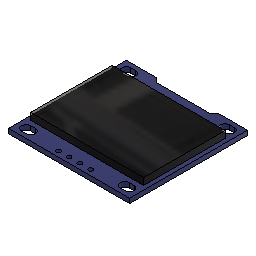
key_emulator (Autodesk Fusion 360 archive; units mm, degrees)
design "OLED Display"
Autodesk Fusion 360 part; units mm, degrees
sketch "Sketch1" plane through (0, 0, 0) normal (0, 1, 0) x (1, 0, 0)
  line L0 (14.25, -13.875) -> (-14.25, -13.875)
  line L1 (-14.25, -13.875) -> (-14.25, 13.875)
  line L2 (14.25, 13.875) -> (14.25, -13.875)
  line L3 (14.25, -13.875) -> (-14.25, 13.875) construction
  line L4 (-14.25, -13.875) -> (14.25, 13.875) construction
  line L5 (-7.25, 13.875) -> (-6.25, 12.875)
  line L6 (-6.25, 12.875) -> (6.25, 12.875)
  line L7 (6.25, 12.875) -> (7.25, 13.875)
  line L8 (-14.25, 13.875) -> (-7.25, 13.875)
  line L9 (7.25, 13.875) -> (14.25, 13.875)
  line L10 (-13.25, -10.725) -> (-10, -10.725)
  line L11 (-10, -10.725) -> (-10, -12.875)
  line L12 (-10, -12.875) -> (-13.25, -12.875)
  line L13 (-13.25, -12.875) -> (-13.25, -10.725)
  line L14 (0, 0) -> (0, -13.875) construction
  line L15 (0, 0) -> (14.25, 0) construction
  line L16 (13.25, -10.725) -> (10, -10.725)
  line L17 (10, -10.725) -> (10, -12.875)
  line L18 (10, -12.875) -> (13.25, -12.875)
  line L19 (13.25, -12.875) -> (13.25, -10.725)
  line L20 (-13.25, 10.725) -> (-10, 10.725)
  line L21 (-10, 12.875) -> (-13.25, 12.875)
  line L22 (10, 12.875) -> (13.25, 12.875)
  line L23 (-13.25, 12.875) -> (-13.25, 10.725)
  line L24 (10, 10.725) -> (10, 12.875)
  line L25 (13.25, 10.725) -> (10, 10.725)
  line L26 (-10, 10.725) -> (-10, 12.875)
  line L27 (13.25, 12.875) -> (13.25, 10.725)
  dimension "d1" = 28.5
  dimension "d2" = 27.75
  dimension "d3" = 135
  dimension "d4" = 7
  dimension "d5" = 7
  dimension "d6" = 1
  dimension "d7" = 3.25
  dimension "d8" = 2.15
  dimension "d9" = 1
  dimension "d10" = 1
  constraint horizontal L0
  constraint perpendicular L0 L1
  constraint parallel L0 L8
  constraint parallel L1 L2
  constraint coincident L3 L14.start
  constraint coincident L4 L14.start
  constraint coincident L14.start L15.start
  constraint parallel L6 L8
  constraint coincident L7.end L8
  constraint perpendicular L5 L7
  constraint collinear L8 L9
  constraint horizontal L10
  constraint vertical L11
  constraint horizontal L12
  constraint vertical L13
  constraint midpoint L0 L14.end
  constraint midpoint L2 L15.end
  constraint symmetric L10.start L14 L16.start
  constraint symmetric L10.end L14 L16.end
  constraint symmetric L11.end L14 L17.end
  constraint symmetric L12.end L14 L18.end
  constraint symmetric L10.start L15 L20.start
  constraint symmetric L10.end L15 L20.end
  constraint symmetric L11.end L15 L21.start
  constraint symmetric L12.end L15 L21.end
  constraint symmetric L15 L17.end L22.start
  constraint symmetric L15 L16.start L25.start
  constraint symmetric L15 L16.end L24.start
  constraint symmetric L15 L18.end L22.end
  measures "d1" distance of L1.end L2.start
  measures "d2" distance of L0.end L1.end
  measures "d3" angle of L5 L6
  measures "d4" distance of L1.end L5.start
  measures "d5" distance of L2.start L7.end
  measures "d6" horizontal distance of L6.end L7.end
  measures "d7" distance of L10.start L10.end
  measures "d8" distance of L10.start L12.end
  measures "d9" distance of L0 L12
  measures "d10" distance of L1 L13
extrude "Extrude1" add sketch "Sketch1" along normal blind 1.1 makes body 1
fillet "Fillet1" radius 1.075 16 edges at (13.25, 0.55, -12.875) (13.25, 0.55, -10.725) (10, 0.55, -10.725) (10, 0.55, -12.875) (-13.25, 0.55, -12.875) (-13.25, 0.55, -10.725) (-10, 0.55, -10.725) (-10, 0.55, -12.875) (-10, 0.55, 10.725) (-13.25, 0.55, 10.725) (-13.25, 0.55, 12.875) (-10, 0.55, 12.875) (13.25, 0.55, 12.875) (10, 0.55, 12.875) (10, 0.55, 10.725) (13.25, 0.55, 10.725) on bodies 1
sketch "Sketch2" plane through (0, 1.1, 0) normal (0, 1, 0) x (-1, 0, 0)
  arc A0 (-12.175, 12.875) -> (-12.175, 10.725) centre (-12.175, 11.8) ccw
  line L0 (-12.175, 12.875) -> (-11.075, 12.875)
  arc A1 (-11.075, 10.725) -> (-11.075, 12.875) centre (-11.075, 11.8) ccw
  line L1 (-11.075, 10.725) -> (-12.175, 10.725)
  line L2 (-11.075, -12.875) -> (-12.175, -12.875)
  arc A2 (-12.175, -10.725) -> (-12.175, -12.875) centre (-12.175, -11.8) ccw
  line L3 (-12.175, -10.725) -> (-11.075, -10.725)
  arc A3 (-11.075, -12.875) -> (-11.075, -10.725) centre (-11.075, -11.8) ccw
  line L4 (11.075, 12.875) -> (12.175, 12.875)
  arc A4 (12.175, 10.725) -> (12.175, 12.875) centre (12.175, 11.8) ccw
  line L5 (12.175, 10.725) -> (11.075, 10.725)
  arc A5 (11.075, 12.875) -> (11.075, 10.725) centre (11.075, 11.8) ccw
  arc A6 (11.075, -10.725) -> (11.075, -12.875) centre (11.075, -11.8) ccw
  line L6 (11.075, -10.725) -> (12.175, -10.725)
  arc A7 (12.175, -12.875) -> (12.175, -10.725) centre (12.175, -11.8) ccw
  line L7 (12.175, -12.875) -> (11.075, -12.875)
  line L8 (-7.25, -13.875) -> (-6.25, -12.875)
  line L9 (-6.25, -12.875) -> (6.25, -12.875)
  line L10 (6.25, -12.875) -> (7.25, -13.875)
  line L11 (7.25, -13.875) -> (14.25, -13.875)
  line L12 (14.25, -13.875) -> (14.25, 13.875)
  line L13 (14.25, 13.875) -> (-14.25, 13.875)
  line L14 (-14.25, 13.875) -> (-14.25, -13.875)
  line L15 (-14.25, -13.875) -> (-7.25, -13.875)
  line L16 (-13.3, 9.625) -> (13.3, 9.625)
  line L17 (13.3, 9.625) -> (13.3, -9.575)
  line L18 (13.3, -9.575) -> (-13.3, -9.575)
  line L19 (-13.3, -9.575) -> (-13.3, 9.625)
  line L20 (-13.3, 9.625) -> (13.3, -9.575) construction
  line L21 (13.3, 9.625) -> (-13.3, -9.575) construction
  point P0 (0, 0.025)
  dimension "d14" = 26.6
  dimension "d15" = 19.2
  dimension "d16" = 4.25
  constraint horizontal L16
  constraint perpendicular L16 L17
  constraint parallel L16 L18
  constraint parallel L17 L19
  constraint coincident L20 P0
  constraint coincident L21 P0
  constraint vertical origin P0
  measures "d14" distance of L17.end L18.end
  measures "d15" distance of L16.end L17.end
  measures "d16" distance of L13 L16
extrude "Extrude2" add sketch "Sketch2" along normal blind 1.6 separate body contours L16 L17 L18 L19 makes body 2
sketch "Sketch3" plane through (0, 1.1, 0) normal (0, 1, 0) x (-1, 0, 0)
  arc A0 (-12.175, 12.875) -> (-12.175, 10.725) centre (-12.175, 11.8) ccw
  line L0 (-12.175, 12.875) -> (-11.075, 12.875)
  arc A1 (-11.075, 10.725) -> (-11.075, 12.875) centre (-11.075, 11.8) ccw
  line L1 (-11.075, 10.725) -> (-12.175, 10.725)
  line L2 (-11.075, -12.875) -> (-12.175, -12.875)
  arc A2 (-12.175, -10.725) -> (-12.175, -12.875) centre (-12.175, -11.8) ccw
  line L3 (-12.175, -10.725) -> (-11.075, -10.725)
  arc A3 (-11.075, -12.875) -> (-11.075, -10.725) centre (-11.075, -11.8) ccw
  line L4 (11.075, 12.875) -> (12.175, 12.875)
  arc A4 (12.175, 10.725) -> (12.175, 12.875) centre (12.175, 11.8) ccw
  line L5 (12.175, 10.725) -> (11.075, 10.725)
  arc A5 (11.075, 12.875) -> (11.075, 10.725) centre (11.075, 11.8) ccw
  arc A6 (11.075, -10.725) -> (11.075, -12.875) centre (11.075, -11.8) ccw
  line L6 (11.075, -10.725) -> (12.175, -10.725)
  arc A7 (12.175, -12.875) -> (12.175, -10.725) centre (12.175, -11.8) ccw
  line L7 (12.175, -12.875) -> (11.075, -12.875)
  line L8 (-7.25, -13.875) -> (-6.25, -12.875)
  line L9 (-6.25, -12.875) -> (6.25, -12.875)
  line L10 (6.25, -12.875) -> (7.25, -13.875)
  line L11 (7.25, -13.875) -> (14.25, -13.875)
  line L12 (14.25, -13.875) -> (14.25, 13.875)
  line L13 (14.25, 13.875) -> (-14.25, 13.875)
  line L14 (-14.25, 13.875) -> (-14.25, -13.875)
  line L15 (-14.25, -13.875) -> (-7.25, -13.875)
  line L16 (5.08, 13.875) -> (2.54, 13.875) construction
  line L17 (2.54, 13.875) -> (2.54, 11.335) construction
  line L18 (2.54, 11.335) -> (5.08, 11.335) construction
  line L19 (5.08, 11.335) -> (5.08, 13.875) construction
  line L20 (5.08, 13.875) -> (2.54, 11.335) construction
  circle A8 centre (3.81, 12.605) radius 0.508
  circle A9 centre (1.27, 12.605) radius 0.508
  circle A10 centre (-1.27, 12.605) radius 0.508
  circle A11 centre (-3.81, 12.605) radius 0.508
  point P0 (0, 13.875)
  point P1 (5.08, 13.875)
  dimension "d28" = 2.54
  dimension "d29" = 2.54
  dimension "d30" = 2.54
  dimension "d31" = 1.016
  dimension "d34" = -7.62
  dimension "d35" = 0
  constraint midpoint L13 P0
  constraint coincident L13 P1
  constraint horizontal L16
  constraint vertical L17
  constraint horizontal L18
  constraint vertical L19
  constraint coincident P1 L16.start
  constraint midpoint L20 A8.centre
  measures "d28" distance of P1 L16.end
  measures "d29" distance of P1 L18.end
  measures "d30" distance of P0 L16.end
  measures "d31" diameter of A8
extrude "Extrude3" cut sketch "Sketch3" against normal through all contours A8 | A9 | A10 | A11 bodies 1
equation "d13 = ( 2.15 / 2 ) * 1 mm"
equation "d34 = ( -2.54 * 3 ) * 1 mm"

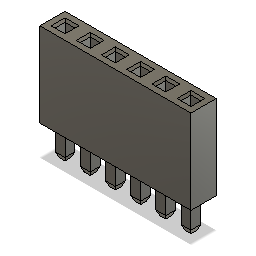
design "Pins"
Autodesk Fusion 360 part; units mm, degrees
sketch "Sketch1" plane through (0, 0, 0) normal (0, 1, 0) x (1, 0, 0)
  line L0 (0, 0) -> (15.24, 0)
  line L1 (15.24, 0) -> (15.24, -2.54)
  line L2 (15.24, -2.54) -> (0, -2.54)
  line L3 (0, -2.54) -> (0, 0)
  line L4 (0, 0) -> (2.54, -2.54) construction
  line L5 (0, 0) -> (3.5921, 0) construction
  line L6 (1.77, -0.77) -> (0.77, -0.77)
  line L7 (0.77, -0.77) -> (0.77, -1.77)
  line L8 (0.77, -1.77) -> (1.77, -1.77)
  line L9 (1.77, -1.77) -> (1.77, -0.77)
  line L10 (1.77, -0.77) -> (0.77, -1.77) construction
  line L11 (0.77, -0.77) -> (1.77, -1.77) construction
  line L12 (4.31, -0.77) -> (3.31, -0.77)
  line L13 (4.31, -0.77) -> (3.31, -1.77) construction
  line L14 (3.31, -1.77) -> (4.31, -1.77)
  line L15 (3.31, -0.77) -> (4.31, -1.77) construction
  line L16 (3.31, -0.77) -> (3.31, -1.77)
  line L17 (4.31, -1.77) -> (4.31, -0.77)
  line L18 (6.85, -0.77) -> (5.85, -0.77)
  line L19 (6.85, -0.77) -> (5.85, -1.77) construction
  line L20 (5.85, -1.77) -> (6.85, -1.77)
  line L21 (5.85, -0.77) -> (6.85, -1.77) construction
  line L22 (5.85, -0.77) -> (5.85, -1.77)
  line L23 (6.85, -1.77) -> (6.85, -0.77)
  line L24 (9.39, -0.77) -> (8.39, -0.77)
  line L25 (9.39, -0.77) -> (8.39, -1.77) construction
  line L26 (8.39, -1.77) -> (9.39, -1.77)
  line L27 (8.39, -0.77) -> (9.39, -1.77) construction
  line L28 (8.39, -0.77) -> (8.39, -1.77)
  line L29 (9.39, -1.77) -> (9.39, -0.77)
  line L30 (11.93, -0.77) -> (10.93, -0.77)
  line L31 (11.93, -0.77) -> (10.93, -1.77) construction
  line L32 (10.93, -1.77) -> (11.93, -1.77)
  line L33 (10.93, -0.77) -> (11.93, -1.77) construction
  line L34 (10.93, -0.77) -> (10.93, -1.77)
  line L35 (11.93, -1.77) -> (11.93, -0.77)
  line L36 (14.47, -0.77) -> (13.47, -0.77)
  line L37 (14.47, -0.77) -> (13.47, -1.77) construction
  line L38 (13.47, -1.77) -> (14.47, -1.77)
  line L39 (13.47, -0.77) -> (14.47, -1.77) construction
  line L40 (13.47, -0.77) -> (13.47, -1.77)
  line L41 (14.47, -1.77) -> (14.47, -0.77)
  point P0 (1.27, -1.27)
  point P1 (3.81, -1.27)
  point P2 (6.35, -1.27)
  point P3 (8.89, -1.27)
  point P4 (11.43, -1.27)
  point P5 (13.97, -1.27)
  dimension "d1" = 15.24
  dimension "d2" = 2.54
  dimension "d3" = 45
  dimension "d4" = 1
  dimension "d5" = 1
  dimension "d8" = 12.7
  dimension "d9" = 0
  constraint horizontal L0
  constraint vertical L1
  constraint horizontal L2
  constraint vertical L3
  constraint coincident L0.start L3.end
  constraint horizontal L5
  constraint coincident L2 L4.end
  constraint horizontal L6
  constraint perpendicular L6 L7
  constraint parallel L6 L8
  constraint parallel L7 L9
  constraint coincident L10 P0
  constraint coincident L11 P0
  constraint midpoint L4 P0
  measures "d1" distance of L1.end L2.end
  measures "d2" distance of L0.end L1.end
  measures "d3" angle of L4 L5
  measures "d4" distance of L7.end L8.end
  measures "d5" distance of L6.end L7.end
extrude "Extrude1" add sketch "Sketch1" along normal blind 8.5 makes body 1
chamfer "Chamfer1" distance 0.2 angle 45 4 edges at (1.77, 8.5, 1.27) (1.27, 8.5, 1.77) (0.77, 8.5, 1.27) (1.27, 8.5, 0.77) on bodies 1
pattern_linear "R-Pattern1" count 6 spacing 2.54 along (1, 0, 0) of "Chamfer1"
ref_plane "WorkPlane1" through (7.62, 4.25, 1.27) normal (0, 0, 1) x (1, 0, 0)
sketch "Sketch2" plane through (7.62, 4.25, 1.27) normal (0, 0, 1) x (1, 0, 0)
  line L0 (-5.85, 4.05) -> (-6.85, 4.05)
  line L1 (-6.85, 4.05) -> (-6.85, -4.25)
  line L2 (-6.85, -4.25) -> (-5.85, -4.25)
  line L3 (-5.85, -4.25) -> (-5.85, 4.05)
  line L4 (-6.85, -4.25) -> (-5.85, -4.25)
  line L5 (-5.85, -4.25) -> (-5.85, -7.25)
  line L6 (-5.85, -7.25) -> (-6.85, -7.25)
  line L7 (-6.85, -7.25) -> (-6.85, -4.25)
  line L8 (-6.85, -4.25) -> (-5.85, -4.25)
  line L9 (-5.85, -4.25) -> (-5.85, -2.75)
  line L10 (-5.85, -2.75) -> (-6.85, -2.75)
  line L11 (-6.85, -2.75) -> (-6.85, -4.25)
  dimension "d18" = 1
  dimension "d19" = 3
  dimension "d20" = 1.5
  constraint horizontal L4
  constraint vertical L5
  constraint horizontal L6
  constraint vertical L7
  constraint coincident L1.end L2.start
  constraint horizontal L8
  constraint vertical L9
  constraint horizontal L10
  constraint vertical L11
  constraint coincident L3 L9.end
  measures "d18" distance of L1.end L2.end
  measures "d19" distance of L1.end L6.end
  measures "d20" distance of L8 L10
extrude "Extrude2" add sketch "Sketch2" along normal mid plane 1 separate body contours L1 L2 L3 L4 L8 L9 L10 L11 | L2 L4 L5 L6 L7 L8 makes body 2
chamfer "Chamfer2" distance 0.5 distance2 0.2 3 edges at (1.27, -3, 1.77) (0.77, -3, 1.27) (1.27, -3, 0.77) measured on face at (1.4367, 0, 1.77) measured on face at (0.77, -1.5, 1.4367) measured on face at (1.4367, 0, 0.77) on bodies 2
chamfer "Chamfer3" distance 0.2 distance2 0.5 1 edges at (1.77, -3, 1.27) measured on face at (1.5033, -3, 1.17) on bodies 2
pattern_linear "R-Pattern2" count 6 spacing 2.54 along (1, 0, 0) of "Extrude2", "Chamfer2", "Chamfer3" makes body 3 at (3.9767, 0.1667, 1.77) makes body 4 at (6.5167, 0.1667, 1.77) makes body 5 at (8.7233, -1.1667, 0.77) makes body 6 at (11.5967, 0.1667, 1.77) makes body 7 at (14.1367, 0.1667, 1.77)
combine "Combine1" operation add target body 1 tool bodies 6 5 3 7 4 2
equation "d1 = ( 2.54 * 6 ) * 1 mm"
equation "d8 = ( 2.54 * 5 ) * 1 mm"
equation "d15 = ( 2.54 * 5 ) * 1 mm"
equation "d17 = ( -2.54 / 2 ) * 1 mm"
equation "d29 = ( 2.54 * 5 ) * 1 mm"

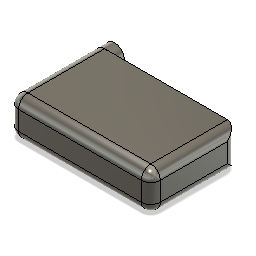
design "JJR 150mah battery"
Autodesk Fusion 360 part; units mm, degrees
sketch "Sketch1" plane through (0, 0, 0) normal (0, 1, 0) x (1, 0, 0)
  line L0 (14, -8.5) -> (-14, -8.5)
  line L1 (-14, -8.5) -> (-14, 8.5)
  line L2 (-14, 8.5) -> (14, 8.5)
  line L3 (14, 8.5) -> (14, -8.5)
  line L4 (14, -8.5) -> (-14, 8.5) construction
  line L5 (-14, -8.5) -> (14, 8.5) construction
  dimension "d1" = 28
  dimension "d2" = 17
  constraint horizontal L0
  constraint perpendicular L0 L1
  constraint parallel L0 L2
  constraint parallel L1 L3
  constraint coincident L4 origin
  constraint coincident L5 origin
  measures "d1" distance of L1.end L2.end
  measures "d2" distance of L0.end L1.end
extrude "Extrude1" add sketch "Sketch1" along normal blind 7.5 makes body 1
sketch "Sketch2" plane through (0, 0, -8.5) normal (0, 0, -1) x (-1, 0, 0)
  line L0 (-14, 0) -> (14, 0)
  line L1 (14, 0) -> (14, 7.5)
  line L2 (14, 7.5) -> (-14, 7.5)
  line L3 (-14, 7.5) -> (-14, 0)
  line L4 (14, 0) -> (6.5, 7.5) construction
  line L5 (14, 7.5) -> (6.5, 0) construction
  line L6 (14, 0) -> (10.25, 3.75) construction
  line L7 (10.25, 3.75) -> (14, 7.5) construction
  circle A0 centre (12.125, 5.625) radius 1.875
  circle A1 centre (12.125, 1.875) radius 1.875
  constraint coincident L0.end L1.start
  constraint coincident L2 L4.end
  constraint coincident L1.end L2.start
  constraint coincident L0 L5.end
  constraint vertical L4.end L5.end
  constraint perpendicular L4 L5
  constraint midpoint L4 L6.end
  constraint midpoint L7 A0.centre
  constraint tangent L1 A0
  constraint midpoint L6 A1.centre
  constraint tangent L1 A1
extrude "Extrude2" add sketch "Sketch2" along normal blind 2 separate body contours A1 | A0 makes body 2
fillet "Fillet1" radius 1.875 9 edges at (-14, 7.5, 0) (14, 3.75, -8.5) (0, 7.5, 8.5) (14, 7.5, 0) (-14, 0, 0) (-14, 3.75, 8.5) (0, 0, 8.5) (14, 3.75, 8.5) (14, 0, 0) on bodies 1
equation "d7 = ( 7.5 / 4 ) * 1 mm"
